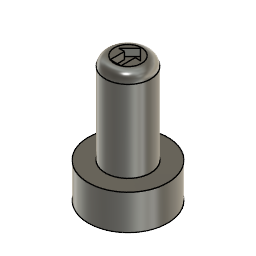
_Button Long.d1430e1f-5d8a-446c-85c3-4e6cc32e4bb1 (Autodesk Fusion 360 design; units mm, degrees)
Autodesk Fusion 360 part; units mm, degrees
sketch "Sketch1" plane through (0, 0, 0) normal (0, 0, 1) x (1, 0, 0)
  line L0 (121.4132, 31.9574) -> (124.1913, 31.9574)
  line L1 (124.1913, 31.9574) -> (124.1913, 29.1793)
  line L2 (124.1913, 29.1793) -> (121.4132, 29.1793)
  line L3 (121.4132, 29.1793) -> (121.4132, 31.9574)
  circle A0 centre (122.8023, 30.5684) radius 5.5563
  dimension "d1" = 2.7781
  dimension "d2" = 2.7781
  dimension "d17" = 11.1125
  constraint horizontal L0
  constraint vertical L1
  constraint horizontal L2
  constraint vertical L3
  measures "d1" distance of L0.start L0.end
  measures "d2" distance of L0.start L2.end
  measures "d17" diameter of A0
extrude "Extrude1" add sketch "Sketch1" along normal blind 2.3813
extrude "Extrude4" add sketch "Sketch1" along normal blind 2.54 from surface at 2.3813 contours L0 L1 L2 L3 | A0
sketch "Sketch2" plane through (0, 0, 4.9213) normal (0, 0, 1) x (-1, 0, 0)
  line L0 (-124.1913, -29.1793) -> (-121.4132, -29.1793)
  line L1 (-121.4132, -29.1793) -> (-121.4132, -31.9574)
  line L2 (-121.4132, -31.9574) -> (-124.1913, -31.9574)
  line L3 (-124.1913, -31.9574) -> (-124.1913, -29.1793)
  circle A0 centre (-122.8023, -30.5684) radius 3.175
  circle A1 centre (-122.8023, -30.5684) radius 5.5562
  circle A2 centre (-122.8023, -30.5684) radius 5.5562
  point P0 (-121.4132, -30.5684)
  point P1 (-122.8023, -31.9574)
  dimension "d6" = 6.35
  constraint midpoint L1 P0
  constraint horizontal A0.centre P0
  constraint midpoint L2 P1
  constraint vertical A0.centre P1
  measures "d6" diameter of A0
extrude "Extrude2" add sketch "Sketch2" along normal blind 12.7 contours L0 L1 L2 L3 | A0
fillet "Fillet1" radius 1.27 1 edges at (125.7624, 31.7165, 17.6213)
sketch "Sketch3" plane through (0, 0, 17.6213) normal (0, 0, 1) x (-1, 0, 0)
  circle A0 centre (-122.8023, -30.5684) radius 1.905
  line L0 (-122.0523, -30.8184) -> (-123.5523, -30.8184) construction
  line L1 (-123.5523, -30.8184) -> (-123.5523, -28.8184)
  line L2 (-123.5523, -28.8184) -> (-122.0523, -28.8184)
  line L3 (-122.0523, -28.8184) -> (-122.0523, -30.8184)
  line L4 (-121.3023, -30.8184) -> (-124.3023, -30.8184)
  line L5 (-124.3023, -30.8184) -> (-122.8023, -32.3184)
  line L6 (-122.8023, -32.3184) -> (-121.3023, -30.8184)
  line L7 (-122.8023, -32.3184) -> (-122.8023, -28.8184) construction
  point P0 (-122.8023, -30.8184)
  point P1 (-122.8023, -30.5684)
  dimension "d11" = 1.5
  dimension "d12" = 2
  dimension "d13" = 1.5
  dimension "d14" = 3
  constraint horizontal L0
  constraint vertical L1
  constraint horizontal L2
  constraint vertical L3
  constraint horizontal L4
  constraint equal L5 L6
  constraint midpoint L0 P0
  constraint vertical L5.end P0
  constraint collinear L0 L4
  constraint midpoint L2 L7.end
  constraint midpoint L7 P1
  constraint coincident A0.centre P1
  measures "d11" distance of L1.end L2.end
  measures "d12" distance of L0.end L1.end
  measures "d13" distance of L4 L5.end
  measures "d14" distance of L4.start L4.end
extrude "Extrude3" cut sketch "Sketch3" against normal blind 1 contours L1 L2 L3 L4 | L4 L5 L6
equation "d1 = ( 7 / 64 ) * 1 in"
equation "d2 = ( 7 / 64 ) * 1 in"
equation "d4 = ( 3 / 32 ) * 1 in"
equation "d17 = ( 7 / 16 ) * 1 in"
